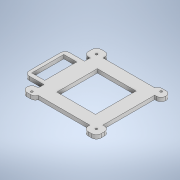
# Autodesk Inventor part: PixfalconHolder
Saved by Autodesk Inventor 2020 (Build 240168000, 168)
## iProperties
Created: 2019-06-13
Part Number: PixfalconHolder
Material: Generic
Document SubType Name: Sheet Metal
Designer: amirt
Density: 1 g/cm^3
Sheet Metal Rule: Default
Appearance: Default
Author: amirt
Autodesk Inventor part; units mm, degrees
ref_plane "YZ Plane" through (0, 0, 0) normal (1, 0, 0) x (0, 1, 0)
ref_plane "XZ Plane" through (0, 0, 0) normal (0, 1, 0) x (-1, 0, 0)
ref_plane "XY Plane" through (0, 0, 0) normal (0, 0, 1) x (1, 0, 0)
sketch "Sketch1" plane through (0, 0, 0) normal (0, 1, 0) x (-1, 0, 0)
  line L0 (42.8447, -6.952) -> (51.5823, -6.952)
  line L1 (51.5823, -6.952) -> (51.5823, -0.4834)
  line L2 (51.5823, -0.4834) -> (42.8447, -0.4834)
  line L3 (42.8447, -0.4834) -> (42.8447, -6.952)
  line L4 (-0.7823, -48.4843) -> (7.9553, -48.4843)
  line L5 (7.9553, -48.4843) -> (7.9553, -42.0157)
  line L6 (7.9553, -42.0157) -> (-0.7823, -42.0157)
  line L7 (-0.7823, -42.0157) -> (-0.7823, -48.4843)
  line L8 (7.9451, -6.952) -> (-0.7823, -6.952)
  line L9 (-0.7823, -6.952) -> (-0.7823, 1.7754)
  line L10 (-0.7823, 1.7754) -> (7.9451, 1.7754)
  line L11 (7.9451, 1.7754) -> (7.9451, -6.952)
  line L12 (42.8549, -50.7432) -> (42.8549, -42.0157)
  line L13 (51.5823, -50.7432) -> (42.8549, -50.7432)
  line L14 (51.5823, -42.0157) -> (51.5823, -50.7432)
  line L15 (42.8549, -42.0157) -> (51.5823, -42.0157)
  line L16 (42.8447, -2.5883) -> (7.935, -2.5883)
  line L17 (42.8549, -42.0157) -> (42.8549, -46.3795)
  line L18 (42.8549, -46.3795) -> (7.9451, -46.3795)
  line L19 (42.8549, -42.0157) -> (47.2186, -42.0157)
  line L20 (7.9451, -6.952) -> (3.5865, -6.952)
  line L21 (3.5865, -6.952) -> (3.5865, -42.0157)
  line L22 (12.309, -38.1974) -> (38.491, -38.1974)
  line L23 (38.491, -38.1974) -> (38.491, -10.7703)
  line L24 (38.491, -10.7703) -> (12.309, -10.7703)
  line L25 (12.309, -10.7703) -> (12.309, -38.1974)
  line L26 (47.2135, -10.7703) -> (60.3097, -10.7703)
  line L27 (60.3097, -10.7703) -> (60.3097, -38.1974)
  line L28 (60.3097, -38.1974) -> (47.2186, -38.1974)
  line L29 (47.2135, -6.952) -> (47.2135, -10.7703)
  line L30 (47.2186, -38.1974) -> (47.2186, -42.0157)
  line L31 (47.2135, -6.952) -> (51.5823, -6.952)
  line L32 (49.4004, -13.4933) -> (58.1279, -13.4933)
  line L33 (58.1279, -13.4933) -> (58.1279, -35.1517)
  line L34 (58.1279, -35.1517) -> (49.4004, -35.1517)
  line L35 (49.4004, -35.1517) -> (49.4004, -13.4933)
  circle A0 centre (47.2186, -2.5883) radius 0.6982
  circle A1 centre (3.5814, -2.5883) radius 0.6982
  circle A2 centre (3.5814, -46.3795) radius 0.6982
  circle A3 centre (47.2186, -46.3795) radius 0.6982
  point P0 (0, 0)
  point P1 (25.4, -24.4839)
  point P2 (3.5865, -6.952)
  point P3 (7.9553, -46.3795)
  point P4 (7.9451, -2.5883)
  point P5 (47.2186, -42.0157)
  dimension "d2" = 8.7376
  dimension "d6" = 360
  dimension "d10" = 360
  dimension "d19" = 5.7909
  dimension "d20" = 5.7909
  dimension "d21" = 13.0912
  dimension "d29" = 1.3964
  dimension "d32" = 360
  dimension "d38" = 43.6372
  constraints: 72 end point, 8 parallel, 6 horizontal, 5 perpendicular, 4 centre point, 3 midpoint, 1 collinear, 1 point on line, 1 vertical, 41 other
  measures "d2" distance of L2.end L1.end
  measures "d19" distance of L0.start L23.end
  measures "d20" distance of L5.end L22.start
  measures "d21" distance of L27.end L28.end
  measures "d29" diameter of A0
  measures "d38" distance of A1.centre A0.centre
extrude "Extrusion3" add sketch "Sketch1" along normal blind 2.54
fillet "Fillet4" radius 3.175 14 edges at (-51.5823, 1.27, -0.4834) (-42.8447, 1.27, -0.4834) (-51.5823, 1.27, -6.952) (-7.9451, 1.27, 1.7754) (0.7823, 1.27, 1.7754) (0.7823, 1.27, -6.952) (0.7823, 1.27, -42.0157) (0.7823, 1.27, -48.4843) (-7.9553, 1.27, -48.4843) (-42.8549, 1.27, -50.7432) (-51.5823, 1.27, -50.7432) (-51.5823, 1.27, -42.0157) (-60.3097, 1.27, -38.1974) (-60.3097, 1.27, -10.7703)
equation "\"BendRadius\" = Thickness"
equation "\"BendReliefWidth\" = Thickness"
equation "\"BendReliefDepth\" = 0.5 * Thickness"
equation "\"CornerReliefSize\" = 4 * Thickness"
equation "\"MinimumRemnant\" = 2 * Thickness"
equation "\"TransitionRadius\" = BendRadius"
equation "\"JacobiRadiusSize\" = BendRadius"
equation "\"GapSize\" = Thickness"
equation "\"Thickness\" = 3.048"
body "Solid3"
